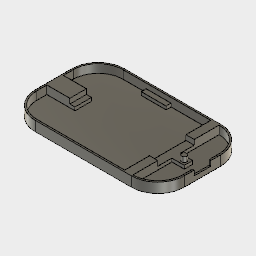
cover_modeling (Autodesk Fusion 360 design; units mm, degrees)
Autodesk Fusion 360 part; units mm, degrees
sketch "Sketch1" plane through (0, 0, 0) normal (0, 0, 1) x (1, 0, 0)
  circle A0 centre (0, 0) radius 25
  line L0 (0, 26) -> (0, 25)
  line L1 (29, 26) -> (-29, 26)
  line L2 (-44, 11) -> (-44, -11)
  line L3 (-29, -26) -> (29, -26)
  line L4 (44, -11) -> (44, 11)
  arc A1 (-29, 26) -> (-44, 11) centre (-29, 11) ccw
  arc A2 (44, 11) -> (29, 26) centre (29, 11) ccw
  arc A3 (-44, -11) -> (-29, -26) centre (-29, -11) ccw
  arc A4 (29, -26) -> (44, -11) centre (29, -11) ccw
  circle A5 centre (34, 0) radius 1.5
  line L5 (-44, 0) -> (-44, 5)
  line L6 (-44, 5) -> (-27, 5)
  line L7 (-27, 5) -> (-27, 0)
  line L8 (-27, 5) -> (-44, 5)
  line L9 (-44, 5) -> (-44, -5)
  line L10 (-44, -5) -> (-27, -5)
  line L11 (-27, -5) -> (-27, 5)
  line L12 (44, 0) -> (25, 0)
  line L13 (0, 26) -> (-15, 26)
  line L14 (-15, 26) -> (-15, 23)
  line L15 (-15, 23) -> (0, 23)
  line L16 (0, 23) -> (0, 26)
  line L17 (0, -26) -> (-15, -26)
  line L18 (-15, -26) -> (-15, -23)
  line L19 (-15, -23) -> (0, -23)
  line L20 (0, -23) -> (0, -26)
  line L21 (29, -26) -> (24, -26)
  line L22 (24, -26) -> (24, 26)
  line L23 (24, 26) -> (29, 26)
  line L24 (29, 26) -> (29, -26)
  line L25 (29, 0) -> (36.5, 0)
  line L26 (36.5, 0) -> (36.5, 2.5)
  line L27 (36.5, 2.5) -> (29, 2.5)
  line L28 (29, 2.5) -> (29, 0)
  line L29 (36.5, 2.5) -> (29, 2.5)
  line L30 (29, 2.5) -> (29, -2.5)
  line L31 (29, -2.5) -> (36.5, -2.5)
  line L32 (36.5, -2.5) -> (36.5, 2.5)
  point P0 (44, 26)
  point P1 (-44, 26)
  point P2 (44, -26)
  dimension "d1" = 50
  dimension "d4" = 26
  dimension "d6" = 52
  dimension "d7" = 88
  dimension "d8" = 15
  dimension "d9" = 15
  dimension "d10" = 15
  dimension "d11" = 15
  dimension "d13" = 3
  dimension "d16" = 5
  dimension "d17" = 10
  dimension "d18" = 3
  dimension "d19" = 15
  dimension "d20" = 15
  dimension "d21" = 3
  dimension "d22" = 52
  dimension "d23" = 5
  dimension "d24" = 2.5
  dimension "d25" = 7.5
  dimension "d26" = 5
  measures "d1" diameter of A0
  measures "d4" distance of A0.centre L0.start
  measures "d6" distance of P0 P2
  measures "d7" distance of P0 P1
  measures "d8" radius of A1
  measures "d9" radius of A2
  measures "d10" radius of A3
  measures "d11" radius of A4
  measures "d13" diameter of A5
  measures "d16" distance of L7.end L6.end
  measures "d17" distance of L6.end L10.end
  measures "d18" distance of L0.start L15.end
  measures "d19" distance of L0.start L13.end
  measures "d20" distance of L17.start L17.end
  measures "d21" distance of L17.start L19.end
  measures "d22" distance of L3.end L1.start
  measures "d23" distance of L3.end L21.end
  measures "d24" distance of L25.start L27.end
  measures "d25" distance of L25.start L25.end
  measures "d26" distance of L26.end L31.end
extrude "Extrude1" add sketch "Sketch1" along normal blind 2 contours A0 L22 | A0 L3 L12 L21 L22 L24 L30 | A0 L1 L12 L22 L23 L24 L28 L30 | A5 L12 L24 L25 L26 L27 L28 L29 L30 L32 | A5 L12 L24 L25 L30 L31 L32 | A0 L15 L16 | A0 L0 L1 L13 L14 L15 L16 | A0 L3 L17 L18 L19 L20 | A0 L19 L20 | A5 L12 L25 | A5 L12 L25 | L2 L5 L6 L7 L8 L9 L10 L11 makes body 1 at (25.6667, -0.8333, 0) makes body 2 at (-10, 24, 0) makes body 3 at (-38.3333, 1.6667, 0) makes body 4 at (-10, -25, 0)
extrude "Extrude2" add sketch "Sketch1" against normal blind 1 bodies 1 2 3 4
sketch "Sketch2" plane through (0, 0, 2) normal (0, 0, 1) x (-1, 0, 0)
  line L0 (-29, 2.5) -> (-36.5, 2.5)
  line L1 (-36.5, 2.5) -> (-36.5, -2.5)
  line L2 (-36.5, -2.5) -> (-29, -2.5)
  line L3 (-29, -2.5) -> (-29, -26)
  line L4 (-29, -26) -> (-24, -26)
  line L5 (-24, -26) -> (-24, 26)
  line L6 (-24, 26) -> (-29, 26)
  line L7 (-29, 26) -> (-29, 2.5)
  circle A0 centre (-34, 0) radius 1.5
extrude "Extrude3" add sketch "Sketch2" along normal blind 3 contours A0 bodies 1
sketch "Sketch3" plane through (0, 0, -1) normal (0, 0, -1) x (1, 0, 0)
  line L0 (-29, -26) -> (29, -26)
  arc A0 (29, -26) -> (44, -11) centre (29, -11) ccw
  line L1 (44, -11) -> (44, 11)
  arc A1 (44, 11) -> (29, 26) centre (29, 11) ccw
  line L2 (29, 26) -> (-29, 26)
  arc A2 (-29, 26) -> (-44, 11) centre (-29, 11) ccw
  line L3 (-44, 11) -> (-44, -11)
  arc A3 (-44, -11) -> (-29, -26) centre (-29, -11) ccw
  arc A4 (-45, -11) -> (-29, -27) centre (-29, -11) ccw
  line L4 (-29, -27) -> (29, -27)
  arc A5 (29, -27) -> (45, -11) centre (29, -11) ccw
  line L5 (45, -11) -> (45, 11)
  arc A6 (45, 11) -> (29, 27) centre (29, 11) ccw
  line L6 (29, 27) -> (-29, 27)
  arc A7 (-29, 27) -> (-45, 11) centre (-29, 11) ccw
  line L7 (-45, 11) -> (-45, -11)
  dimension "d33" = 1
extrude "Extrude4" add sketch "Sketch3" against normal blind 6 bodies 1
sketch "Sketch4" plane through (45, 0, 0) normal (1, 0, 0) x (0, 1, 0)
  line L0 (-11, -1) -> (11, -1)
  line L1 (11, -1) -> (11, 5)
  line L2 (11, 5) -> (-11, 5)
  line L3 (-11, 5) -> (-11, -1)
  line L4 (0, 5) -> (5, 5)
  line L5 (5, 5) -> (5, 2)
  line L6 (5, 2) -> (0, 2)
  line L7 (0, 2) -> (0, 5)
  line L8 (5, 5) -> (-5, 5)
  line L9 (-5, 5) -> (-5, 2)
  line L10 (-5, 2) -> (5, 2)
  line L11 (5, 2) -> (5, 5)
  dimension "d36" = 5
  dimension "d37" = 3
  dimension "d38" = 10
  measures "d36" distance of L4.start L4.end
  measures "d37" distance of L4.start L6.end
  measures "d38" distance of L4.end L8.end
extrude "Extrude5" cut sketch "Sketch4" against normal blind 2 contours L2 L7 L8 L9 L10 | L2 L4 L5 L6 L7 L8 L10 L11 bodies 1
move_body "Move1" bodies 1 to x (1, 0, 0) y (0, 1, 0) z (0, 0, 1) at (0, 0, 1)
sketch "Sketch5" plane through (0, 0, 3) normal (0, 0, 1) x (-1, 0, 0)
  line L0 (27, 5) -> (27, -5)
  line L1 (27, -5) -> (44, -5)
  line L2 (44, -5) -> (44, 5)
  line L3 (44, 5) -> (27, 5)
  line L4 (44, -5) -> (30.1, -5)
  line L5 (30.1, -5) -> (30.1, 5)
  line L6 (30.1, 5) -> (44, 5)
  line L7 (44, 5) -> (44, -5)
  dimension "d41" = 13.9
  measures "d41" distance of L1.end L4.end
extrude "Extrude6" add sketch "Sketch5" along normal blind 3 contours L1 L2 L3 L4 L5 L6 L7 bodies 1
sketch "Sketch6" plane through (0, 0, 3) normal (0, 0, 1) x (-1, 0, 0)
  circle A0 centre (-34, 0) radius 1.5
  line L0 (-29, 2.5) -> (-36.5, 2.5)
  line L1 (-36.5, 2.5) -> (-36.5, -2.5)
  line L2 (-36.5, -2.5) -> (-29, -2.5)
  line L3 (-29, -2.5) -> (-29, -26)
  line L4 (-29, -26) -> (-24, -26)
  line L5 (-24, -26) -> (-24, 26)
  line L6 (-24, 26) -> (-29, 26)
  line L7 (-29, 26) -> (-29, 2.5)
  line L8 (-29, -26) -> (-24, -26)
  line L9 (-24, -26) -> (-24, -11)
  line L10 (-24, -11) -> (-29, -11)
  line L11 (-29, -11) -> (-29, -26)
  line L12 (-29, 26) -> (-24, 26)
  line L13 (-24, 26) -> (-24, 11)
  line L14 (-24, 11) -> (-29, 11)
  line L15 (-29, 11) -> (-29, 26)
  dimension "d44" = 15
  dimension "d45" = 15
  measures "d44" distance of L3.end L10.end
  measures "d45" distance of L6.end L14.end
extrude "Extrude7" add sketch "Sketch6" along normal blind 3 contours L5 L6 L7 L12 L13 L14 L15 | L3 L4 L5 L8 L9 L10 L11 bodies 1
